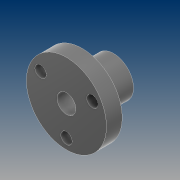
# Autodesk Inventor part: Nakretka_prowadnica_tloka
Saved by Autodesk Inventor 2021 (Build 250183000, 183)
## iProperties
Created: 2022-10-06
Part Number: Nakretka_prowadnica_tloka
Material: Generic
Document SubType Name: Modeling
Designer: agnpi
Density: 1 g/cm^3
Appearance: Smooth - Black
Author: agnpi
Autodesk Inventor part; units mm, degrees
ref_plane "YZ Plane" through (0, 0, 0) normal (1, 0, 0) x (0, 1, 0)
ref_plane "XZ Plane" through (0, 0, 0) normal (0, 1, 0) x (-1, 0, 0)
ref_plane "XY Plane" through (0, 0, 0) normal (0, 0, 1) x (1, 0, 0)
sketch "Sketch1" plane through (0, 0, 0) normal (0, 0, 1) x (1, 0, 0)
  line L0 (-17.85, 0) -> (17.85, 0) construction
  line L1 (0, -17.85) -> (0, 17.85) construction
  circle A0 centre (0, 0) radius 12.75
  dimension "d0" = 25.5
  constraints: 1 centre point, 1 coincident
  measures "d0" diameter of A0
extrude "Extrusion1" add sketch "Sketch1" along normal blind 5
sketch "Sketch2" plane through (0, 0, 0) normal (0, 0, -1) x (-1, 0, 0)
  circle A0 centre (0, 0) radius 6.35
  dimension "d3" = 12.7
  constraints: 1 centre point, 1 coincident
  measures "d3" diameter of A0
extrude "Extrusion2" add sketch "Sketch2" along normal blind 10
sketch "Sketch3" plane through (0, 0, -10) normal (0, 0, -1) x (-1, 0, 0)
  circle A0 centre (0, 0) radius 3
  dimension "d6" = 6
  constraints: 1 centre point, 1 coincident
  measures "d6" diameter of A0
extrude "Extrusion3" cut sketch "Sketch3" against normal through all
sketch "Sketch5" plane through (0, 0, 5) normal (0, 0, 1) x (1, 0, 0)
  circle A0 centre (0, 0) radius 9.525 construction
  circle A1 centre (0, -9.525) radius 1.8
  line L0 (-17.85, 0) -> (17.85, 0) construction
  line L1 (0, -17.85) -> (0, 17.85) construction
  circle A2 centre (8.2489, 4.7625) radius 1.8
  circle A3 centre (-8.2489, 4.7625) radius 1.8
  dimension "d13" = 19.05
  dimension "d14" = 3.6
  dimension "d19" = 360
  constraints: 3 centre point, 1 coincident, 1 point on line, 1 vertical alignment, 9 other
  measures "d14" diameter of A1
extrude "Extrusion5" cut sketch "Sketch5" against normal through all
body "Solid1"
